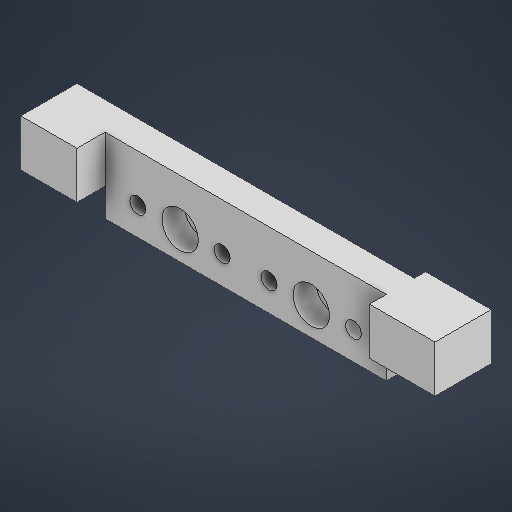
# Autodesk Inventor part: lmwall
Saved by Autodesk Inventor 2026.2 (Build 302298010, 298A)
## iProperties
Created: 2026-04-27
Part Number: lmwall
Material: Ogólny
Document SubType Name: Modeling
Designer: karol
Density: 1 g/cm^3
Appearance: Domyślna
Mass: 0.908014 g
Surface Area: 11.1465 cm^2
Volume: 0.908014 cm^3
Author: karol
Autodesk Inventor part; units mm, degrees
ref_plane "YZ Plane" through (0, 0, 0) normal (1, 0, 0) x (0, 1, 0)
ref_plane "XZ Plane" through (0, 0, 0) normal (0, 1, 0) x (-1, 0, 0)
ref_plane "XY Plane" through (0, 0, 0) normal (0, 0, 1) x (1, 0, 0)
sketch "Szkic1" plane through (0, 0, 0) normal (0, 1, 0) x (-1, 0, 0)
  line L0 (0, 0) -> (42, 0)
  line L1 (42, 0) -> (42, -3)
  line L2 (42, -3) -> (0, -3)
  line L3 (0, -3) -> (0, 0)
  dimension "d0" = 42
  dimension "d1" = 3
  constraints: 8 end point, 2 parallel, 1 horizontal, 1 perpendicular
  measures "d0" distance of L1.end L2.end
  measures "d1" distance of L0.end L1.end
extrude "Wyciągnięcie proste1" add sketch "Szkic1" along normal blind 8
sketch "Szkic2" plane through (0, 8, 0) normal (0, 1, 0) x (1, 0, 0)
  circle A0 centre (-38.7043, 1.357) radius 1
  point P0 (0, 0)
  dimension "d4" = 2
  constraints: 1 centre point
  measures "d4" diameter of A0
extrude "Wyciągnięcie proste2" cut sketch "Szkic2" against normal blind 0.2
sketch "Szkic3" plane through (-42, 0, 0) normal (0, 0, 1) x (1, 0, 0)
  line L0 (0, 8) -> (42, 8) projected
  line L1 (0, 8) -> (6, 8)
  line L2 (6, 0) -> (0, 0)
  line L3 (0, 0) -> (0, 8)
  line L4 (42, 0) -> (36, 0)
  line L5 (36, 8) -> (42, 8)
  line L6 (42, 8) -> (42, 0)
  circle A0 centre (9.5, 3) radius 0.85
  line L7 (0, 0) -> (42, 0) projected
  circle A1 centre (18.5, 3) radius 0.85
  circle A2 centre (23.5, 3) radius 0.85
  circle A3 centre (32.5, 3) radius 0.85
  circle A4 centre (14, 3) radius 1.95
  circle A5 centre (28, 3) radius 1.95
  dimension "d7" = 6
  dimension "d8" = 8
  dimension "d9" = 6
  dimension "d10" = 1.7
  dimension "d11" = 3
  dimension "d12" = 1.7
  dimension "d13" = 1.7
  dimension "d14" = 1.7
  dimension "d15" = 3
  dimension "d16" = 3
  dimension "d17" = 3
  dimension "d18" = 9.5
  dimension "d19" = 9.5
  dimension "d20" = 9
  dimension "d21" = 9
  dimension "d22" = 3.9
  dimension "d23" = 3.9
  dimension "d24" = 3
  dimension "d25" = 4.5
  dimension "d26" = 4.5
  dimension "d27" = 3
  constraints: 12 end point, 6 centre point, 2 horizontal, 2 parallel, 1 point on line
  measures "d7" distance of L2.start L2.end
  measures "d8" distance of L1.end L2.start
  measures "d9" distance of L5.start L5.end
  measures "d10" diameter of A0
  measures "d11" distance from line of L7 A0.centre
  measures "d12" diameter of A1
  measures "d13" diameter of A2
  measures "d14" diameter of A3
  measures "d15" distance from line of L7 A1.centre
  measures "d16" distance from line of L7 A2.centre
  measures "d17" distance from line of L7 A3.centre
  measures "d18" distance from line of L3 A0.centre
  measures "d19" distance from line of L6 A3.centre
  measures "d20" distance of A2.centre A3.centre
  measures "d21" distance of A0.centre A1.centre
  measures "d22" diameter of A4
  measures "d23" diameter of A5
  measures "d24" distance from line of L7 A5.centre
  measures "d25" distance of A5.centre A3.centre
  measures "d26" distance of A0.centre A4.centre
  measures "d27" distance from line of L7 A4.centre
extrude "Wyciągnięcie proste3" cut sketch "Szkic3" against normal blind 3 contours A0 | A1 | A2 | A3 | A4 | A5
sketch "Szkic4" plane through (0, 8, 0) normal (0, 1, 0) x (1, 0, 0)
  line L0 (0, 3) -> (-42, 3) projected
  line L1 (-42, 3) -> (-36, 3)
  line L2 (-36, 3) -> (-36, -3)
  line L3 (-36, -3) -> (-42, -3)
  line L4 (-42, -3) -> (-42, 3)
  point P0 (0, 0)
  dimension "d30" = 6
  dimension "d31" = 6
  constraints: 8 end point, 2 parallel, 1 horizontal, 1 perpendicular
  measures "d30" distance of L2.end L3.end
  measures "d31" distance of L1.end L2.end
extrude "Wyciągnięcie proste4" add sketch "Szkic4" against normal blind 8
sketch "Szkic5" plane through (0, 0, 0) normal (0, -1, 0) x (1, 0, 0)
  line L0 (-36, 3) -> (-42, 3) projected
  line L1 (-42, -3) -> (-36, -3)
  line L2 (-36, -3) -> (-36, 3)
  line L3 (-36, 3) -> (-42, 3)
  line L4 (-42, 3) -> (-42, -3)
  point P0 (0, 0)
  constraints: 8 end point, 2 parallel, 1 horizontal, 1 perpendicular
extrude "Wyciągnięcie proste5" cut sketch "Szkic5" against normal blind 3
sketch "Szkic6" plane through (0, 3, 0) normal (0, -1, 0) x (1, 0, 0)
  circle A0 centre (-39, 0) radius 2
  line L0 (-42, 3) -> (-36, 3) projected
  line L1 (-42, -3) -> (-42, 3) projected
  point P0 (0, 0)
  point P1 (-42, 0)
  dimension "d36" = 4
  dimension "d37" = 3
  dimension "d38" = 3
  constraints: 1 centre point, 1 midpoint
  measures "d36" diameter of A0
  measures "d37" distance from line of L0 A0.centre
  measures "d38" distance of point (-42, 0) A0.centre
extrude "Wyciągnięcie proste6" cut sketch "Szkic6" against normal blind 4
sketch "Szkic10" plane through (0, 8, 0) normal (0, 1, 0) x (1, 0, 0)
  line L0 (0, 3) -> (-36, 3) projected
  line L1 (0, 3) -> (-6, 3)
  line L2 (-6, 3) -> (-6, -1.8)
  line L3 (-6, -1.8) -> (0, -1.8)
  line L4 (0, -1.8) -> (0, 3)
  line L5 (-6, 3) -> (0, 3)
  line L6 (0, 3) -> (0, 4.2)
  line L7 (0, 4.2) -> (-6, 4.2)
  line L8 (-6, 4.2) -> (-6, 3)
  line L9 (0, 4.2) -> (1, 4.2)
  line L10 (1, 4.2) -> (1, -1.8)
  line L11 (1, -1.8) -> (0, -1.8)
  line L12 (0, -1.8) -> (0, 4.2)
  point P0 (0, 0)
  dimension "d55" = 6
  dimension "d56" = 4.8
  dimension "d57" = 1.2
  dimension "d58" = 1
  constraints: 24 end point, 6 parallel, 3 horizontal, 3 perpendicular, 1 point on line
  measures "d55" distance of L3.end L2.end
  measures "d56" distance of L2.end L1.end
  measures "d57" distance of L6.end L5.end
  measures "d58" distance of L10.end L11.end
extrude "Wyciągnięcie proste10" add sketch "Szkic10" against normal blind 8
sketch "Szkic11" plane through (0, 0, 0) normal (0, -1, 0) x (1, 0, 0)
  line L0 (-6, 1.8) -> (1, 1.8) projected
  line L1 (-6, -3) -> (-6, -4.2) projected
  line L2 (1, 1.8) -> (-6, 1.8)
  line L3 (-6, 1.8) -> (-6, -4.2)
  line L4 (-6, -4.2) -> (1, -4.2)
  line L5 (1, -4.2) -> (1, 1.8)
  point P0 (0, 0)
  constraints: 8 end point, 2 parallel, 1 horizontal, 1 perpendicular
extrude "Wyciągnięcie proste11" cut sketch "Szkic11" against normal blind 3
sketch "Szkic12" plane through (0, 3, 0) normal (0, -1, 0) x (1, 0, 0)
  circle A0 centre (-2, -1.2) radius 2
  line L0 (1, 1.8) -> (1, -4.2) projected
  line L1 (-6, -3) -> (-6, 0) projected
  line L2 (-6, 1.8) -> (1, 1.8) projected
  point P0 (0, 0)
  point P1 (1, -1.2)
  point P2 (-6, -1.5)
  dimension "d63" = 4
  dimension "d64" = 3
  dimension "d65" = 4
  dimension "d66" = 3
  constraints: 2 midpoint, 1 centre point
  measures "d63" diameter of A0
  measures "d64" distance of point (1, -1.2) A0.centre
  measures "d65" horizontal distance of point (-6, -1.5) A0.centre
  measures "d66" distance from line of L2 A0.centre
extrude "Wyciągnięcie proste12" cut sketch "Szkic12" against normal blind 3.25
sketch "Szkic14" plane through (-36, 3, -3) normal (0, 0, -1) x (-1, 0, 0)
  circle A0 centre (-22, 0) radius 1.95 projected
  circle A1 centre (-22, 0) radius 2.2
  circle A2 centre (-8, 0) radius 1.95 projected
  circle A3 centre (-8, 0) radius 2.2
  point P0 (-36, -3)
  dimension "d73" = 4.4
  dimension "d74" = 4.4
  constraints: 2 centre point, 2 coincident
  measures "d73" diameter of A1
  measures "d74" diameter of A3
extrude "Wyciągnięcie proste14" cut sketch "Szkic14" against normal blind 0.6 contours A0 | A1 | A2 | A3
